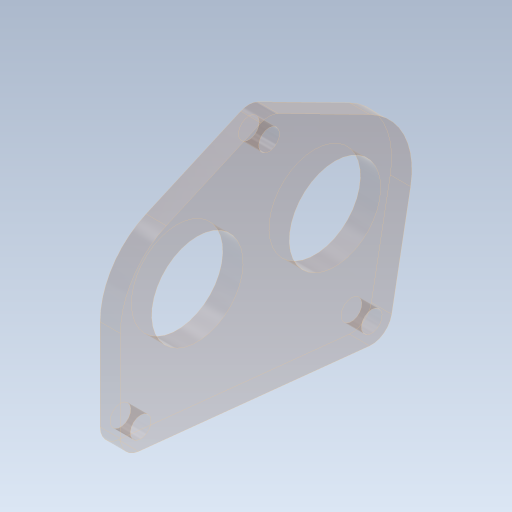
# Autodesk Inventor part: INDX_012_OuterPlate
Saved by Autodesk Inventor 2024 (Build 280153000, 153)
## iProperties
Created: 2024-07-27
Part Number: INDX_012_OuterPlate
Material: Polycarbonate, Smoke
Document SubType Name: Modeling
Designer: Oscar
Density: 1.2 g/cm^3
Appearance: Polycarbonate - Smoked
Author: Oscar
Autodesk Inventor part; units mm, degrees
ref_plane "YZ Plane" through (0, 0, 0) normal (1, 0, 0) x (0, 1, 0)
ref_plane "XZ Plane" through (0, 0, 0) normal (0, 1, 0) x (-1, 0, 0)
ref_plane "XY Plane" through (0, 0, 0) normal (0, 0, 1) x (1, 0, 0)
sketch "Sketch1" plane through (0, 0, 0) normal (1, 0, 0) x (0, 1, 0)
  line L0 (95.25, 812.8) -> (44.45, 812.8) construction
  line L1 (44.45, 812.8) -> (44.45, 0) construction
  line L2 (44.45, 0) -> (95.25, 0) construction
  line L3 (95.25, 0) -> (95.25, 812.8) construction
  line L4 (95.25, 0) -> (44.45, 0) construction
  line L5 (44.45, 25.4) -> (95.25, 25.4) construction
  circle A0 centre (190.5, 0) radius 50.8 construction
  circle A1 centre (95.25, 279.4) radius 25.4 construction
  circle A2 centre (274.9493, 279.9916) radius 9.525 construction
  circle A3 centre (274.9493, 279.9916) radius 25.4 construction
  circle A4 centre (274.9493, 279.9916) radius 31.75 construction
  circle A5 centre (609.6, 438.15) radius 50.8 construction
  circle A6 centre (274.9493, 279.9916) radius 30.48 construction
  circle A7 centre (587.8333, 365.125) radius 25.4 construction
  circle A8 centre (587.8333, 511.175) radius 25.4 construction
  line L6 (587.8333, 485.775) -> (587.8333, 390.525) construction
  circle A9 centre (490.3356, 512.7625) radius 14.351 construction
  circle A10 centre (392.825, 512.7625) radius 14.351 construction
  circle A11 centre (490.3356, 363.5375) radius 14.351 construction
  line L7 (587.8333, 511.175) -> (490.3356, 512.7625) construction
  line L8 (587.8333, 365.125) -> (490.3356, 363.5375) construction
  circle A12 centre (490.3356, 512.7625) radius 25.4 construction
  circle A13 centre (490.3356, 363.5375) radius 25.4 construction
  line L9 (490.3356, 487.3625) -> (490.3356, 388.9375) construction
  circle A14 centre (392.825, 512.7625) radius 25.4 construction
  circle A15 centre (392.825, 363.5375) radius 25.4 construction
  circle A16 centre (392.825, 363.5375) radius 14.351 construction
  line L10 (490.3356, 512.7625) -> (392.825, 512.7625) construction
  line L11 (490.3356, 363.5375) -> (392.825, 363.5375) construction
  line L12 (392.825, 487.3625) -> (392.825, 388.9375) construction
  circle A17 centre (295.3189, 511.8309) radius 25.4 construction
  circle A18 centre (295.3189, 362.6059) radius 25.4 construction
  circle A19 centre (203.1597, 479.9719) radius 25.4 construction
  circle A20 centre (295.3189, 511.8309) radius 14.351 construction
  circle A21 centre (295.3189, 362.6059) radius 14.351 construction
  circle A22 centre (203.1597, 479.9719) radius 14.351 construction
  line L13 (392.825, 512.7625) -> (295.3189, 511.8309) construction
  line L14 (392.825, 363.5375) -> (295.3189, 362.6059) construction
  line L15 (295.3189, 486.4309) -> (295.3189, 388.0059) construction
  line L16 (295.3189, 511.8309) -> (203.1597, 479.9719) construction
  circle A23 centre (123.1487, 424.2353) radius 25.4 construction
  circle A24 centre (123.1487, 424.2353) radius 14.351 construction
  line L17 (203.1597, 479.9719) -> (123.1487, 424.2353) construction
  circle A25 centre (95.25, 279.4) radius 14.351 construction
  line L18 (609.6, 355.6) -> (44.45, 355.6) construction
  line L19 (44.45, 355.6) -> (44.45, 330.2) construction
  line L20 (44.45, 330.2) -> (609.6, 330.2) construction
  line L21 (609.6, 330.2) -> (609.6, 355.6) construction
  line L22 (95.25, 241.3) -> (44.45, 241.3) construction
  line L23 (44.45, 241.3) -> (44.45, 215.9) construction
  line L24 (44.45, 215.9) -> (95.25, 215.9) construction
  line L25 (95.25, 215.9) -> (95.25, 241.3) construction
  circle A26 centre (244.475, 279.4) radius 25.4 construction
  circle A27 centre (244.475, 279.4) radius 14.351 construction
  line L26 (218.8463, 459.9947) -> (279.6322, 382.5831) construction
  circle A28 centre (274.9493, 279.9916) radius 8.89 construction
  circle A29 centre (288.401, 252.6405) radius 21.59 construction
  circle A30 centre (244.475, 279.4) radius 21.59 construction
  circle A31 centre (288.401, 252.6405) radius 14.351
  circle A32 centre (587.8333, 511.175) radius 14.351 construction
  circle A33 centre (587.8333, 365.125) radius 14.351 construction
  line L27 (95.25, 647.7) -> (609.6, 647.7) construction
  line L28 (609.6, 647.7) -> (609.6, 622.3) construction
  line L29 (609.6, 622.3) -> (95.25, 622.3) construction
  line L30 (95.25, 622.3) -> (95.25, 647.7) construction
  circle A34 centre (600.5333, 552.45) radius 3.2639 construction
  circle A35 centre (600.5333, 552.45) radius 6.35 construction
  circle A36 centre (600.5333, 336.55) radius 3.2639 construction
  circle A37 centre (600.5333, 336.55) radius 6.35 construction
  circle A38 centre (114.3, 552.45) radius 3.2639 construction
  circle A39 centre (114.3, 552.45) radius 6.35 construction
  line L31 (595.3031, 535.4518) -> (598.6659, 546.3808) construction
  circle A40 centre (63.5, 264.8503) radius 3.2639 construction
  circle A41 centre (63.5, 264.8503) radius 6.35 construction
  line L32 (337.9424, 330.2) -> (600.5333, 330.2) construction
  circle A42 centre (288.401, 252.6405) radius 24.13 construction
  circle A43 centre (244.475, 279.4) radius 24.13 construction
  line L33 (72.1591, 268.8184) -> (69.2727, 267.4957) construction
  line L34 (609.6, 342.9) -> (44.45, 342.9) construction
  line L35 (265.0822, 266.8462) -> (267.7937, 265.1944) construction
  circle A44 centre (318.8924, 273.2978) radius 3.2639
  circle A45 centre (253.4257, 241.1003) radius 3.2639
  line L36 (95.25, 558.8) -> (44.45, 558.8) construction
  line L37 (44.45, 558.8) -> (44.45, 533.4) construction
  line L38 (44.45, 533.4) -> (95.25, 533.4) construction
  line L39 (95.25, 533.4) -> (95.25, 558.8) construction
  line L40 (114.3, 558.8) -> (600.5333, 558.8) construction
  line L41 (108.0468, 553.5545) -> (57.2468, 265.9549) construction
  line L42 (285.1949, 228.7245) -> (62.6563, 258.5566) construction
  circle A46 centre (318.8924, 273.2978) radius 6.35 construction
  circle A47 centre (253.4257, 241.1003) radius 6.35 construction
  arc A48 (114.3, 558.8) -> (108.0468, 553.5545) centre (114.3, 552.45) ccw construction
  arc A49 (57.2468, 265.9549) -> (62.6563, 258.5566) centre (63.5, 264.8503) ccw construction
  line L43 (312.6148, 274.2541) -> (306.3372, 275.2103) construction
  line L44 (313.6352, 269.7362) -> (308.3781, 266.1746) construction
  line L45 (259.4559, 243.09) -> (265.4861, 245.0797) construction
  line L46 (256.5005, 246.6562) -> (259.5753, 252.2121) construction
  line L47 (325.2424, 317.5) -> (325.2424, 273.2978) construction
  arc A50 (337.9424, 330.2) -> (325.2424, 317.5) centre (337.9424, 317.5) ccw construction
  line L48 (324.5494, 270.4133) -> (309.8976, 241.6792) construction
  arc A51 (324.5494, 270.4133) -> (325.2424, 273.2978) centre (318.8924, 273.2978) ccw construction
  arc A52 (285.1949, 228.7245) -> (309.8976, 241.6792) centre (288.401, 252.6405) ccw construction
  circle A53 centre (431.8, 342.9) radius 3.2639 construction
  circle A54 centre (457.2, 342.9) radius 3.2639 construction
  circle A55 centre (520.7, 342.9) radius 3.2639 construction
  circle A56 centre (546.1, 342.9) radius 3.2639 construction
  line L49 (606.8833, 552.45) -> (606.8833, 336.55) construction
  arc A57 (606.8833, 552.45) -> (600.5333, 558.8) centre (600.5333, 552.45) ccw construction
  arc A58 (600.5333, 330.2) -> (606.8833, 336.55) centre (600.5333, 336.55) ccw construction
  circle A59 centre (184.15, 304.8) radius 3.2639 construction
  circle A60 centre (158.75, 304.8) radius 3.2639 construction
  circle A61 centre (133.35, 304.8) radius 3.2639 construction
  circle A62 centre (133.35, 279.4) radius 3.2639 construction
  circle A63 centre (158.75, 279.4) radius 3.2639 construction
  circle A64 centre (184.15, 279.4) radius 3.2639 construction
  circle A65 centre (289.5545, 295.8051) radius 21.59 construction
  line L50 (313.8542, 277.163) -> (306.6842, 282.6636) construction
  circle A66 centre (289.5545, 295.8051) radius 14.351
  circle A67 centre (260.9795, 313.5851) radius 3.2639
  circle A68 centre (260.9795, 313.5851) radius 6.35 construction
  circle A69 centre (289.5545, 295.8051) radius 24.13 construction
  line L51 (266.371, 310.2304) -> (269.0668, 308.553) construction
  line L52 (252.257, 234.8587) -> (283.9601, 228.9227)
  line L53 (324.5494, 270.4133) -> (309.8976, 241.6792)
  arc A70 (283.9601, 228.9227) -> (309.8976, 241.6792) centre (288.401, 252.6405) ccw
  line L54 (247.1099, 241.7584) -> (254.6637, 314.2433)
  line L55 (260.9795, 319.9351) -> (289.5545, 319.9351)
  line L56 (324.7039, 275.8568) -> (311.6384, 305.5292)
  arc A71 (311.6384, 305.5292) -> (289.5545, 319.9351) centre (289.5545, 295.8051) ccw
  arc A72 (324.5494, 270.4133) -> (324.7039, 275.8568) centre (318.8924, 273.2978) ccw
  arc A73 (260.9795, 319.9351) -> (254.6637, 314.2433) centre (260.9795, 313.5851) ccw
  arc A74 (247.1099, 241.7584) -> (252.257, 234.8587) centre (253.4257, 241.1003) ccw
  point P0 (0, 0)
  point P1 (241.139, 234.6303)
  point P2 (100.4185, 253.4945)
  dimension "d9" = 50.8
  dimension "d38" = 50.8
  dimension "d53" = 50.8
  dimension "d178" = 43.18
  dimension "d1" = 812.8
  dimension "d2" = 44.45
  dimension "d4" = 25.4
  dimension "d5" = 101.6
  dimension "d6" = 95.25
  dimension "d8" = 50.8
  dimension "d14" = 50.8
  dimension "d15" = 63.5
  dimension "d21" = 19.05
  dimension "d29" = 438.15
  dimension "d30" = 514.35
  dimension "d36" = 60.96
  dimension "d39" = 50.8
  dimension "d41" = 95.25
  dimension "d45" = 28.702
  dimension "d47" = 97.5106
  dimension "d48" = 98.425
  dimension "d56" = 25.4
  dimension "d73" = 50.8
  dimension "d74" = 25.4
  dimension "d75" = 215.9
  dimension "d78" = 279.4
  dimension "d80" = 149.225
  dimension "d81" = 97.5106
  dimension "d82" = 147.4978
  dimension "d83" = 17.78
  dimension "d85" = 43.18
  dimension "d92" = 330.2
  dimension "d100" = 514.35
  dimension "d107" = 25.4
  dimension "d108" = 514.35
  dimension "d109" = 266.7
  dimension "d115" = 6.5278
  dimension "d116" = 12.7
  dimension "d122" = 2.54
  dimension "d123" = 2.54
  dimension "d128" = 3.175
  dimension "d134" = 3.175
  dimension "d135" = 194.9958
  dimension "d136" = 6.5278
  dimension "d137" = 25.4
  dimension "d138" = 533.4
  dimension "d139" = 19.05
  dimension "d140" = 19.05
  dimension "d141" = 12.7
  dimension "d142" = 6.35
  dimension "d143" = 12.7
  dimension "d144" = 43.18
  dimension "d149" = 25.4
  dimension "d151" = 6.5278
  dimension "d157" = 25.4
  dimension "d158" = 63.5
  dimension "d159" = 12.7
  dimension "d161" = 11.4347
  dimension "d163" = 44.45
  dimension "d164" = 38.1
  dimension "d166" = 336.55
  dimension "d167" = 25.4
  dimension "d168" = 6.5278
  dimension "d169" = 25.4
  dimension "d170" = 25.4
  dimension "d173" = 25.4
  dimension "d174" = 38.1
  dimension "d175" = 25.4
  constraints: 112 end point, 63 centre point, 51 point on circle, 36 point on line, 29 equal radius, 27 coincident, 24 tangent, 12 equal length, 10 parallel, 9 horizontal, 9 horizontal alignment, 9 vertical alignment, 5 concentric, 5 perpendicular, 5 vertical, 2 midpoint, 65 other
  measures "d1" distance of L1.end L0.end
  measures "d2" distance from line of point (0, 0) L1
  measures "d4" distance of L4.end L5.start
  measures "d5" diameter of A0
  measures "d14" diameter of A3
  measures "d15" diameter of A4
  measures "d21" diameter of A2
  measures "d29" distance from line of L2 point (609.6, 438.15)
  measures "d36" diameter of A6
  measures "d39" diameter of A8
  measures "d41" distance of L6.start L6.end
  measures "d45" diameter of A9
  measures "d47" distance of L7.start L7.end
  measures "d48" distance of L9.start L9.end
  measures "d56" distance of L20.end L18.start
  measures "d73" distance of L24.end L23.end
  measures "d74" distance of L23.end L22.end
  measures "d75" distance between parallel lines of L2 L24
  measures "d78" distance from line of L2 point (95.25, 279.4)
  measures "d80" distance of point (95.25, 279.4) A26.centre
  measures "d81" distance of A26.centre A18.centre
  measures "d82" distance of point (95.25, 279.4) A23.centre
  measures "d83" diameter of A28
  measures "d85" diameter of A29
  measures "d92" distance between parallel lines of L2 L20
  measures "d107" distance between parallel lines of L29 L27
  measures "d108" distance of L28.end L29.end
  measures "d109" distance between parallel lines of L18 L29
  measures "d115" diameter of A34
  measures "d116" diameter of A35
  measures "d128" distance of L33.start L33.end
  measures "d134" distance of L35.start L35.end
  measures "d135" distance of A25.centre A31.centre
  measures "d136" diameter of A45
  measures "d137" distance between parallel lines of L36 L38
  measures "d138" distance between parallel lines of L2 L38
  measures "d140" distance from line of L1 A40.centre
  measures "d141" diameter of A47
  measures "d142" distance of L44.start L44.end
  measures "d143" radius of A50
  measures "d144" diameter of A30
  measures "d149" distance of A53.centre A54.centre
  measures "d151" diameter of A53
  measures "d157" distance of A56.centre A55.centre
  measures "d158" distance of A54.centre A55.centre
  measures "d159" horizontal distance of L7.start A35.centre
  measures "d161" distance of L31.start L31.end
  measures "d163" distance of L42.start point (241.139, 234.63)
  measures "d164" distance of L42.end point (100.419, 253.494)
  measures "d167" distance between parallel lines of L2 L5
  measures "d168" diameter of A59
  measures "d169" distance of A59.centre A60.centre
  measures "d170" distance of A61.centre A60.centre
  measures "d173" distance from line of A61.centre L20
  measures "d175" distance of A63.centre A60.centre
extrude "Extrusion2" add sketch "Sketch1" along normal blind 6.35
body "Solid2"
